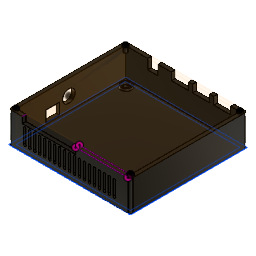
ControllerCaseLower (Autodesk Fusion 360 design; units mm, degrees)
Autodesk Fusion 360 part; units mm, degrees
sketch "Sketch1" plane through (0, 0, 0) normal (0, 0, 1) x (1, 0, 0)
  line L0 (-99.906, 117.6419) -> (-1.906, 117.6419)
  line L1 (-1.906, 117.6419) -> (-1.906, 23.6419)
  line L2 (-1.906, 23.6419) -> (-99.906, 23.6419)
  line L3 (-99.906, 23.6419) -> (-99.906, 117.6419)
  line L4 (-96.906, 114.6419) -> (-4.906, 114.6419)
  line L5 (-4.906, 114.6419) -> (-4.906, 26.6419)
  line L6 (-4.906, 26.6419) -> (-96.906, 26.6419)
  line L7 (-96.906, 26.6419) -> (-96.906, 114.6419)
  dimension "d1" = 98
  dimension "d2" = 94
  dimension "d3" = 92
  dimension "d4" = 88
  dimension "d5" = 3
  dimension "d6" = 3
  constraint horizontal L0
  constraint vertical L1
  constraint horizontal L2
  constraint vertical L3
  constraint horizontal L4
  constraint vertical L5
  constraint horizontal L6
  constraint vertical L7
  measures "d1" distance of L0.start L0.end
  measures "d2" distance of L0.start L2.end
  measures "d3" distance of L4.start L4.end
  measures "d4" distance of L4.start L6.end
  measures "d5" distance of L0 L4
  measures "d6" distance of L3 L7
extrude "Extrude1" add sketch "Sketch1" along normal blind 2 contours L0 L1 L2 L3 | L4 L5 L6 L7 makes body 1
sketch "Sketch2" plane through (0, 0, 2) normal (0, 0, 1) x (-1, 0, 0)
  line L0 (99.906, -23.6419) -> (1.906, -23.6419)
  line L1 (1.906, -23.6419) -> (1.906, -117.6419)
  line L2 (1.906, -117.6419) -> (99.906, -117.6419)
  line L3 (99.906, -117.6419) -> (99.906, -23.6419)
  line L4 (90.406, -108.6419) -> (13.406, -108.6419) construction
  line L5 (13.406, -108.6419) -> (13.406, -32.6419) construction
  line L6 (13.406, -32.6419) -> (90.406, -32.6419) construction
  line L7 (90.406, -32.6419) -> (90.406, -108.6419) construction
  circle A0 centre (90.406, -108.6419) radius 4
  circle A1 centre (13.406, -108.6419) radius 4
  circle A2 centre (13.406, -32.6419) radius 4
  circle A3 centre (90.406, -32.6419) radius 4
  circle A4 centre (90.406, -108.6419) radius 3
  circle A5 centre (13.406, -108.6419) radius 3
  circle A6 centre (13.406, -32.6419) radius 3
  circle A7 centre (90.406, -32.6419) radius 3
  dimension "d9" = 77
  dimension "d10" = 76
  dimension "d11" = 11.5
  dimension "d12" = 9
  dimension "d13" = 8
  dimension "d14" = 8
  dimension "d15" = 8
  dimension "d16" = 8
  dimension "d20" = 6
  dimension "d21" = 6
  dimension "d22" = 6
  dimension "d23" = 6
  constraint horizontal L4
  constraint vertical L5
  constraint horizontal L6
  constraint vertical L7
  constraint coincident L4.start L7.end
  constraint coincident L4.end L5.start
  constraint coincident L5.end L6.start
  constraint coincident L6.end L7.start
  measures "d9" distance of L4.start L4.end
  measures "d10" distance of L4.start L6.end
  measures "d11" distance of L1 L5
  measures "d12" distance of L2 L4
  measures "d13" diameter of A0
  measures "d14" diameter of A1
  measures "d15" diameter of A2
  measures "d16" diameter of A3
  measures "d20" diameter of A4
  measures "d21" diameter of A5
  measures "d22" diameter of A6
  measures "d23" diameter of A7
hole "Hole1" at (-90.406, 32.6419, 2) at (-90.406, 108.6419, 2) at (-13.406, 108.6419, 2) at (-13.406, 32.6419, 2) direction (0, 0, -1) diameter 5.5 depth 3 tip angle 118 bodies 1
extrude "Extrude2" add sketch "Sketch2" along normal blind 2 contours A0 | A1 | A2 | A3 bodies 1
extrude "Extrude3" add sketch "Sketch1" along normal blind 25 bodies 1
sketch "Sketch3" plane through (-96.906, 0, 0) normal (1, 0, 0) x (0, 1, 0)
  line L0 (26.6419, 2) -> (114.6419, 2)
  line L1 (114.6419, 2) -> (114.6419, 25)
  line L2 (114.6419, 25) -> (26.6419, 25)
  line L3 (26.6419, 25) -> (26.6419, 2)
  line L4 (50.6419, 3) -> (61.6419, 3)
  line L5 (61.6419, 3) -> (61.6419, 12)
  line L6 (61.6419, 12) -> (50.6419, 12)
  line L7 (50.6419, 12) -> (50.6419, 3)
  circle A0 centre (69.1419, 12.5) radius 5
  dimension "d30" = 11
  dimension "d31" = 9
  dimension "d32" = 1
  dimension "d35" = 53
  dimension "d52" = 10
  dimension "d53" = 10.5
  dimension "d54" = 45.5
  constraint horizontal L4
  constraint vertical L5
  constraint horizontal L6
  constraint vertical L7
  measures "d30" distance of L4.start L4.end
  measures "d31" distance of L4.start L6.end
  measures "d32" distance of L0 L4
  measures "d35" distance of L1 L5
  measures "d52" diameter of A0
  measures "d53" distance of L0 A0.centre
  measures "d54" distance of L1 A0.centre
extrude "Extrude4" cut sketch "Sketch3" against normal blind 4 contours L4 L5 L6 L7 | A0 bodies 1
sketch "Sketch4" plane through (0, 26.6419, 0) normal (0, 1, 0) x (-1, 0, 0)
  line L0 (4.906, 2) -> (96.906, 2)
  line L1 (96.906, 2) -> (96.906, 25)
  line L2 (96.906, 25) -> (4.906, 25)
  line L3 (4.906, 25) -> (4.906, 2)
  line L4 (13.906, 6) -> (13.906, 18)
  arc A0 (15.906, 18) -> (13.906, 18) centre (14.906, 18) ccw
  line L5 (15.906, 18) -> (15.906, 6)
  arc A1 (13.906, 6) -> (15.906, 6) centre (14.906, 6) ccw
  arc A2 (19.906, 18) -> (17.906, 18) centre (18.906, 18) ccw
  arc A3 (17.906, 6) -> (19.906, 6) centre (18.906, 6) ccw
  line L6 (17.906, 6) -> (17.906, 18)
  line L7 (19.906, 18) -> (19.906, 6)
  arc A4 (23.906, 18) -> (21.906, 18) centre (22.906, 18) ccw
  arc A5 (21.906, 6) -> (23.906, 6) centre (22.906, 6) ccw
  line L8 (21.906, 6) -> (21.906, 18)
  line L9 (23.906, 18) -> (23.906, 6)
  arc A6 (27.906, 18) -> (25.906, 18) centre (26.906, 18) ccw
  arc A7 (25.906, 6) -> (27.906, 6) centre (26.906, 6) ccw
  line L10 (25.906, 6) -> (25.906, 18)
  line L11 (27.906, 18) -> (27.906, 6)
  arc A8 (31.906, 18) -> (29.906, 18) centre (30.906, 18) ccw
  arc A9 (29.906, 6) -> (31.906, 6) centre (30.906, 6) ccw
  line L12 (29.906, 6) -> (29.906, 18)
  line L13 (31.906, 18) -> (31.906, 6)
  arc A10 (35.906, 18) -> (33.906, 18) centre (34.906, 18) ccw
  arc A11 (33.906, 6) -> (35.906, 6) centre (34.906, 6) ccw
  line L14 (33.906, 6) -> (33.906, 18)
  line L15 (35.906, 18) -> (35.906, 6)
  arc A12 (39.906, 18) -> (37.906, 18) centre (38.906, 18) ccw
  arc A13 (37.906, 6) -> (39.906, 6) centre (38.906, 6) ccw
  line L16 (37.906, 6) -> (37.906, 18)
  line L17 (39.906, 18) -> (39.906, 6)
  arc A14 (43.906, 18) -> (41.906, 18) centre (42.906, 18) ccw
  arc A15 (41.906, 6) -> (43.906, 6) centre (42.906, 6) ccw
  line L18 (41.906, 6) -> (41.906, 18)
  line L19 (43.906, 18) -> (43.906, 6)
  arc A16 (47.906, 18) -> (45.906, 18) centre (46.906, 18) ccw
  arc A17 (45.906, 6) -> (47.906, 6) centre (46.906, 6) ccw
  line L20 (45.906, 6) -> (45.906, 18)
  line L21 (47.906, 18) -> (47.906, 6)
  arc A18 (51.906, 18) -> (49.906, 18) centre (50.906, 18) ccw
  arc A19 (49.906, 6) -> (51.906, 6) centre (50.906, 6) ccw
  line L22 (49.906, 6) -> (49.906, 18)
  line L23 (51.906, 18) -> (51.906, 6)
  arc A20 (55.906, 18) -> (53.906, 18) centre (54.906, 18) ccw
  arc A21 (53.906, 6) -> (55.906, 6) centre (54.906, 6) ccw
  line L24 (53.906, 6) -> (53.906, 18)
  line L25 (55.906, 18) -> (55.906, 6)
  arc A22 (59.906, 18) -> (57.906, 18) centre (58.906, 18) ccw
  arc A23 (57.906, 6) -> (59.906, 6) centre (58.906, 6) ccw
  line L26 (57.906, 6) -> (57.906, 18)
  line L27 (59.906, 18) -> (59.906, 6)
  arc A24 (63.906, 18) -> (61.906, 18) centre (62.906, 18) ccw
  arc A25 (61.906, 6) -> (63.906, 6) centre (62.906, 6) ccw
  line L28 (61.906, 6) -> (61.906, 18)
  line L29 (63.906, 18) -> (63.906, 6)
  arc A26 (67.906, 18) -> (65.906, 18) centre (66.906, 18) ccw
  arc A27 (65.906, 6) -> (67.906, 6) centre (66.906, 6) ccw
  line L30 (65.906, 6) -> (65.906, 18)
  line L31 (67.906, 18) -> (67.906, 6)
  arc A28 (71.906, 18) -> (69.906, 18) centre (70.906, 18) ccw
  arc A29 (69.906, 6) -> (71.906, 6) centre (70.906, 6) ccw
  line L32 (69.906, 6) -> (69.906, 18)
  line L33 (71.906, 18) -> (71.906, 6)
  arc A30 (75.906, 18) -> (73.906, 18) centre (74.906, 18) ccw
  arc A31 (73.906, 6) -> (75.906, 6) centre (74.906, 6) ccw
  line L34 (73.906, 6) -> (73.906, 18)
  line L35 (75.906, 18) -> (75.906, 6)
  arc A32 (79.906, 18) -> (77.906, 18) centre (78.906, 18) ccw
  arc A33 (77.906, 6) -> (79.906, 6) centre (78.906, 6) ccw
  line L36 (77.906, 6) -> (77.906, 18)
  line L37 (79.906, 18) -> (79.906, 6)
  arc A34 (83.906, 18) -> (81.906, 18) centre (82.906, 18) ccw
  arc A35 (81.906, 6) -> (83.906, 6) centre (82.906, 6) ccw
  line L38 (81.906, 6) -> (81.906, 18)
  line L39 (83.906, 18) -> (83.906, 6)
  arc A36 (87.906, 18) -> (85.906, 18) centre (86.906, 18) ccw
  arc A37 (85.906, 6) -> (87.906, 6) centre (86.906, 6) ccw
  line L40 (85.906, 6) -> (85.906, 18)
  line L41 (87.906, 18) -> (87.906, 6)
  line L42 (45.906, 25) -> (88.906, 25)
  line L43 (88.906, 25) -> (88.906, 20)
  line L44 (88.906, 20) -> (45.906, 20)
  line L45 (45.906, 20) -> (45.906, 25)
  line L46 (1.906, 0) -> (99.906, 0)
  dimension "d42" = 2
  dimension "d43" = 12
  dimension "d44" = 9
  dimension "d47" = 4
  dimension "d48" = 0
  dimension "d77" = 43
  dimension "d78" = 5
  dimension "d80" = 4
  dimension "d82" = 8
  constraint vertical L4
  constraint tangent L4 A0
  constraint tangent A0 L5
  constraint parallel L4 L5
  constraint tangent L5 A1
  constraint tangent L4 A1
  constraint horizontal L42
  constraint vertical L43
  constraint horizontal L44
  constraint vertical L45
  constraint coincident L2 L42.start
  measures "d42" distance of L4 L5
  measures "d43" distance of A0.centre A1.centre
  measures "d44" distance of L3 L4
  measures "d77" distance of L42.start L42.end
  measures "d78" distance of L42.start L44.end
  measures "d80" distance of L0 A1.centre
  measures "d82" distance of L1 L43
extrude "Extrude6" cut sketch "Sketch4" against normal blind 10 contours L2 L42 L43 L44 L45 | L4 A0 L5 A1 | A2 A3 L6 L7 | A4 A5 L8 L9 | A6 A7 L10 L11 | A8 A9 L12 L13 | A10 A11 L14 L15 | A12 A13 L16 L17 | A14 A15 L18 L19 | A16 A17 L20 L21 | A18 A19 L22 L23 | A20 A21 L24 L25 | A22 A23 L26 L27 | A24 A25 L28 L29 | A26 A27 L30 L31 | A28 A29 L32 L33 | A30 A31 L34 L35 | A32 A33 L36 L37 | A34 A35 L38 L39 | A36 A37 L40 L41 bodies 1
fillet "Fillet1" radius 2 4 edges at (-99.906, 23.6419, 12.5) (-99.906, 117.6419, 12.5) (-1.906, 23.6419, 12.5) (-1.906, 117.6419, 12.5) on bodies 1
sketch "Sketch5" plane through (0, 0, 25) normal (0, 0, 1) x (-1, 0, 0)
  line L0 (4.906, -26.6419) -> (96.906, -26.6419)
  line L1 (96.906, -26.6419) -> (96.906, -114.6419)
  line L2 (96.906, -114.6419) -> (4.906, -114.6419)
  line L3 (4.906, -114.6419) -> (4.906, -26.6419)
  arc A0 (1.906, -115.6419) -> (3.906, -117.6419) centre (3.906, -115.6419) ccw
  line L4 (3.906, -117.6419) -> (97.906, -117.6419)
  arc A1 (97.906, -117.6419) -> (99.906, -115.6419) centre (97.906, -115.6419) ccw
  line L5 (99.906, -115.6419) -> (99.906, -25.6419)
  arc A2 (99.906, -25.6419) -> (97.906, -23.6419) centre (97.906, -25.6419) ccw
  line L6 (97.906, -23.6419) -> (88.906, -23.6419)
  arc A3 (3.906, -23.6419) -> (1.906, -25.6419) centre (3.906, -25.6419) ccw
  line L7 (1.906, -25.6419) -> (1.906, -115.6419)
  circle A4 centre (4.906, -114.6419) radius 2
  circle A5 centre (96.906, -114.6419) radius 2
  circle A6 centre (96.906, -26.6419) radius 2
  circle A7 centre (4.906, -26.6419) radius 2
  line L8 (88.906, -23.6419) -> (88.906, -26.6419)
  line L9 (4.906, -26.6419) -> (45.906, -26.6419)
  line L10 (45.906, -26.6419) -> (45.906, -23.6419)
  line L11 (45.906, -23.6419) -> (3.906, -23.6419)
  dimension "d61" = 4
  dimension "d62" = 4
  dimension "d63" = 4
  dimension "d64" = 4
  constraint coincident L2.end L3.start
  constraint coincident L1.end L2.start
  constraint coincident L0.end L1.start
  constraint coincident L0.start L3.end
  measures "d61" diameter of A5
  measures "d62" diameter of A4
  measures "d63" diameter of A7
  measures "d64" diameter of A6
extrude "Extrude7" add sketch "Sketch5" against normal blind 4 contours L0 L3 A7 L9 | L2 L3 A4 | L0 L1 A6 | L1 L2 A5 picked at (6.1521, -27.1067) picked at (6.2326, -114.5471) picked at (95.9656, -27.5823) picked at (95.5795, -114.5471) bodies 1
hole "Hole2" at (-96.906, 26.6419, 25) at (-96.906, 114.6419, 25) at (-4.906, 26.6419, 25) at (-4.906, 114.6419, 25) direction (0, 0, -1) diameter 2.5 depth 4 tip angle 118 bodies 1
copy_body "Body->Comp1" bodies 1 removing the originals makes body 2 in component "Component"
sketch "Sketch6" plane through (0, 117.6419, 0) normal (0, 1, 0) x (-1, 0, 0)
  line L0 (3.906, 25) -> (3.906, 0)
  line L1 (3.906, 0) -> (97.906, 0)
  line L2 (97.906, 0) -> (97.906, 25)
  line L3 (97.906, 25) -> (3.906, 25)
  line L4 (12.406, 25) -> (25.906, 25)
  line L5 (25.906, 25) -> (25.906, 19)
  line L6 (25.906, 19) -> (12.406, 19)
  line L7 (12.406, 19) -> (12.406, 25)
  line L8 (1.906, 25) -> (1.906, 0)
  line L9 (42.906, 25) -> (42.906, 19)
  line L10 (42.906, 19) -> (29.406, 19)
  line L11 (29.406, 19) -> (29.406, 25)
  line L12 (29.406, 25) -> (42.906, 25)
  line L13 (59.906, 25) -> (59.906, 19)
  line L14 (59.906, 19) -> (46.406, 19)
  line L15 (46.406, 19) -> (46.406, 25)
  line L16 (46.406, 25) -> (59.906, 25)
  line L17 (70.906, 25) -> (78.906, 25)
  line L18 (78.906, 25) -> (78.906, 17)
  line L19 (78.906, 17) -> (70.906, 17)
  line L20 (70.906, 17) -> (70.906, 25)
  line L21 (99.906, 0) -> (99.906, 25)
  dimension "d65" = 13.5
  dimension "d66" = 6
  dimension "d67" = 10.5
  dimension "d70" = 17
  dimension "d71" = 0
  dimension "d72" = 8
  dimension "d73" = 8
  dimension "d74" = 21
  constraint horizontal L4
  constraint vertical L5
  constraint horizontal L6
  constraint vertical L7
  constraint coincident L3 L4.start
  constraint horizontal L17
  constraint vertical L18
  constraint horizontal L19
  constraint vertical L20
  constraint coincident L3 L17.start
  measures "d65" distance of L5 L7
  measures "d66" distance of L4 L6
  measures "d67" distance of L7 L8
  measures "d72" distance of L17.start L17.end
  measures "d73" distance of L17.start L19.end
  measures "d74" distance of L18 L21
extrude "Extrude1'" cut sketch "Sketch6" against normal blind 6 contours L3 L4 L5 L6 L7 | L3 L9 L10 L11 L12 | L3 L17 L18 L19 L20 | L3 L13 L14 L15 L16 bodies 2 in component "Component"
component "Component" placed x (1, 0, 0) y (0, 1, 0) z (0, 0, 1) at (0, 0, 0)
